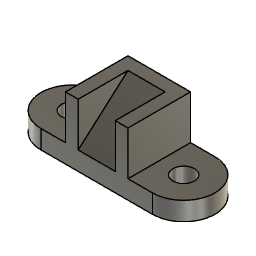
A2 (Autodesk Fusion 360 design; units mm, degrees)
Autodesk Fusion 360 part; units mm, degrees
note: some values were not read from the file. Chosen so that the rebuilt part matches the saved one: which pieces of a blend or face edit are solid.
sketch "Sketch1" plane through (0, 0, 0) normal (0, 0, 1) x (1, 0, 0)
  line L0 (-35, 25) -> (143, 25)
  line L1 (143, 25) -> (143, -39)
  line L2 (143, -39) -> (-35, -39)
  line L3 (-35, -39) -> (-35, 25)
  dimension "d1" = 178
  dimension "d2" = 64
  constraint horizontal L0
  constraint vertical L1
  constraint horizontal L2
  constraint vertical L3
  measures "d1" distance of L0.start L0.end
  measures "d2" distance of L0.start L2.end
extrude "Extrude1" add sketch "Sketch1" along normal blind 19
fillet "Fillet1" radius 32 1 faces at (143, 3.6667, 6.3333)
fillet "Fillet2" radius 32 1 faces at (-35, -17.6667, 6.3333)
sketch "Sketch2" plane through (0, 0, 19) normal (0, 0, 1) x (-1, 0, 0)
  arc A0 (3, -25) -> (3, 39) centre (3, 7) ccw
  line L0 (3, 39) -> (-111, 39)
  arc A1 (-111, 39) -> (-111, -25) centre (-111, 7) ccw
  line L1 (-111, -25) -> (3, -25)
  line L2 (-54, -25) -> (-86, -25)
  line L3 (-86, -25) -> (-86, 39)
  line L4 (-86, 39) -> (-54, 39)
  line L5 (-54, 39) -> (-54, -25)
  line L6 (-54, -25) -> (-22, -25)
  line L7 (-22, -25) -> (-22, 39)
  line L8 (-22, 39) -> (-54, 39)
  line L9 (-54, 39) -> (-54, -25)
  line L10 (-54, 39) -> (-54, -12)
  line L11 (-54, -12) -> (-73, -12)
  line L12 (-73, -12) -> (-73, 39.6926)
  line L13 (-73, 39.6926) -> (-54, 39.6926)
  line L14 (-54, 39.6926) -> (-54, -12)
  line L15 (-54, -12) -> (-35, -12)
  line L16 (-35, -12) -> (-35, 39)
  line L17 (-35, 39) -> (-54, 39)
  line L18 (-54, 39) -> (-54, -12)
  dimension "d9" = 32
  dimension "d10" = 64
  dimension "d11" = 32
  dimension "d12" = 51
  dimension "d13" = 19
  dimension "d14" = 19
  constraint horizontal L2
  constraint vertical L3
  constraint horizontal L4
  constraint vertical L5
  constraint midpoint L1 L2.start
  constraint horizontal L6
  constraint vertical L7
  constraint horizontal L8
  constraint vertical L9
  constraint coincident L0 L7.end
  constraint coincident L9 L10.end
  constraint horizontal L11
  constraint vertical L12
  constraint horizontal L13
  constraint vertical L14
  constraint horizontal L15
  constraint vertical L16
  constraint horizontal L17
  constraint vertical L18
  measures "d9" distance of L2.start L2.end
  measures "d10" distance of L2.start L4.end
  measures "d11" distance of L2.start L6.end
  measures "d12" distance of L4.end L10.end
  measures "d13" distance of L10.end L11.end
  measures "d14" distance of L10.end L15.end
extrude "Extrude2" add sketch "Sketch2" along normal blind 45 contours L0 L1 L5 L6 L7 L8 L9 L15 L16 | L0 L1 L2 L3 L4 L5 L9 L11 L12
sketch "Sketch3" plane through (35, 0, 0) normal (1, 0, 0) x (0, 1, 0)
  line L0 (-39, 19) -> (12, 19)
  line L1 (12, 19) -> (12, 64)
  line L2 (12, 64) -> (-39, 64)
  line L3 (-39, 64) -> (-39, 19)
  line L4 (12, 19) -> (-39, 19)
  line L5 (12, 64) -> (12, 19)
  line L6 (12, 64) -> (-39, 19)
  constraint coincident L0.end L1.start
  constraint coincident L0.start L3.end
  constraint coincident L1.end L2.start
extrude "Extrude3" add sketch "Sketch3" along normal blind 38 contours L0 L1 L4 L5 L6
sketch "Sketch4" plane through (0, 0, 19) normal (0, 0, 1) x (-1, 0, 0)
  line L0 (-86, -25) -> (-86, 39)
  line L1 (-86, 39) -> (-111, 39)
  arc A0 (-111, 39) -> (-111, -25) centre (-111, 7) ccw
  line L2 (-111, -25) -> (-86, -25)
  circle A1 centre (-111, 7) radius 11
  dimension "d19" = 22
  constraint concentric A0 A1
  measures "d19" diameter of A1
hole "Hole1" at (111, -7, 19) direction (0, 0, -1) diameter 22 depth 50 tip angle 118
sketch "Sketch5" plane through (0, 0, 19) normal (0, 0, 1) x (-1, 0, 0)
  line L0 (-22, 39) -> (-22, -25)
  line L1 (-22, -25) -> (3, -25)
  arc A0 (3, -25) -> (3, 39) centre (3, 7) ccw
  line L2 (3, 39) -> (-22, 39)
  circle A1 centre (3, 7) radius 11
  dimension "d23" = 22
  constraint concentric A0 A1
  measures "d23" diameter of A1
hole "Hole2" at (-3, -7, 19) direction (0, 0, -1) diameter 22 depth 50 tip angle 118
